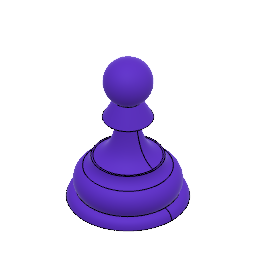
Team Prop - Blue (Autodesk Fusion 360 design; units mm, degrees)
Autodesk Fusion 360 part; units mm, degrees
sketch "Sketch1" plane through (0, 0, 0) normal (0, 0, 1) x (1, 0, 0)
  line L0 (0, 0) -> (38.1, 0)
  line L1 (0, 0) -> (0, 101.6)
  spline S0 degree 5 poles (38.1, 0) (38.0729, 0.2251) (38.0107, 0.6676) (37.894, 1.3084) (37.6903, 2.1164) (37.3503, 3.0435) (36.9172, 3.8802) (36.383, 4.6188) (35.743, 5.2549) (35.0009, 5.7918) (34.1642, 6.2369) (33.4251, 6.5253) (32.8341, 6.7061) (32.4241, 6.811) (32.2151, 6.8596) knots 0 0 0 0 0 0 0.1 0.2 0.3 0.4 0.5 0.6 0.7 0.8 0.9 1 1 1 1 1 1
  arc A0 (32.2151, 6.8596) -> (27.94, 22.86) centre (22.8566, 12.9305) ccw
  arc A1 (22.86, 30.48) -> (27.94, 22.86) centre (32.2172, 31.2148) ccw
  line L2 (22.86, 30.48) -> (21.6124, 30.48)
  line L3 (8.8369, 72.5369) -> (15.9847, 59.2957)
  line L4 (15.9847, 59.2957) -> (7.2582, 59.2957)
  arc A2 (8.8369, 72.5369) -> (0, 101.6) centre (0, 85.725) ccw
  spline S1 degree 5 poles (21.6124, 30.48) (21.0949, 30.6834) (20.0823, 31.124) (18.6306, 31.8864) (16.8317, 33.1096) (14.8242, 35.0045) (13.0719, 37.2921) (11.5828, 39.9944) (10.3418, 43.1067) (9.3177, 46.6065) (8.4762, 50.4692) (7.9246, 53.8339) (7.5695, 56.5069) (7.3578, 58.3551) (7.2582, 59.2957) knots 0 0 0 0 0 0 0.1 0.2 0.3 0.4 0.5 0.6 0.7 0.8 0.9 1 1 1 1 1 1
  line L5 (7.7519, 54.6333) -> (6.7645, 63.9581)
  point P0 (36.3193, 4.6365)
  point P1 (12.7, 38.1)
  dimension "d1" = 38.1
  dimension "d2" = 101.6
  dimension "d4" = 31.75
  constraint coincident L0.start L1.start
  constraint horizontal L0
  constraint perpendicular L0 L1
  constraint tangent A0 A1
  constraint perpendicular L1 L2
  constraint coincident L2 S1.start
  constraint perpendicular L1 L4
  constraint midpoint L4.end L5
  constraint coincident S1 L2.end
  measures "d1" distance of L0.start L0.end
  measures "d2" distance of L0.start L1.end
  measures "d4" diameter of A2
revolve "Revolve1" add sketch "Sketch1" angle 360 about axis through (0, 0, 0) along (0, 1, 0)
